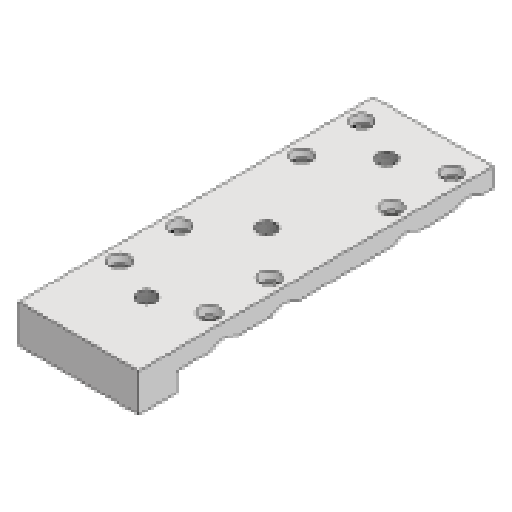
# Autodesk Inventor part: Carrige Attatchment
Saved by Autodesk Inventor 2023 (Build 270158000, 158)
## iProperties
Created: 2022-11-02
Part Number: Carrige Attatchment
Material: Generic
Document SubType Name: Modeling
Designer: deli
Density: 1 g/cm^3
Appearance: Default
Author: deli
Autodesk Inventor part; units mm, degrees
ref_plane "YZ Plane" through (0, 0, 0) normal (1, 0, 0) x (0, 1, 0)
ref_plane "XZ Plane" through (0, 0, 0) normal (0, 1, 0) x (-1, 0, 0)
ref_plane "XY Plane" through (0, 0, 0) normal (0, 0, 1) x (1, 0, 0)
sketch "Sketch1" plane through (0, 0, 0) normal (0, 1, 0) x (-1, 0, 0)
  line L0 (12.8211, 54.4482) -> (-7.1789, 54.4482)
  line L1 (-7.1789, 54.4482) -> (-7.1789, -4.7018)
  line L2 (-7.1789, -4.7018) -> (12.8211, -4.7018)
  line L3 (12.8211, -4.7018) -> (12.8211, 54.4482)
  circle A0 centre (10.3211, 38.6482) radius 1.6
  circle A1 centre (10.3211, 28.6482) radius 1.6
  circle A2 centre (-4.6789, 38.6482) radius 1.6
  circle A3 centre (-4.6789, 28.6482) radius 1.6
  line L4 (10.3211, 38.6482) -> (10.3211, 28.6482) construction
  line L5 (10.3211, 28.6482) -> (-4.6789, 28.6482) construction
  line L6 (-4.6789, 28.6482) -> (-4.6789, 38.6482) construction
  line L7 (-4.6789, 38.6482) -> (10.3211, 38.6482) construction
  circle A4 centre (10.3211, 9.7482) radius 1.6
  circle A5 centre (10.3211, -0.2518) radius 1.6
  circle A6 centre (-4.6789, 9.7482) radius 1.6
  circle A7 centre (-4.6789, -0.2518) radius 1.6
  line L8 (10.3211, 9.7482) -> (10.3211, -0.2518) construction
  line L9 (10.3211, -0.2518) -> (-4.6789, -0.2518) construction
  line L10 (-4.6789, -0.2518) -> (-4.6789, 9.7482) construction
  line L11 (-4.6789, 9.7482) -> (10.3211, 9.7482) construction
  circle A8 centre (2.8211, 43.0982) radius 1.5
  circle A9 centre (2.8211, 23.0982) radius 1.5
  circle A10 centre (2.8211, 3.0982) radius 1.5
  line L12 (2.8211, 43.0982) -> (2.8211, 3.0982) construction
  point P0 (0, 0)
  dimension "d0" = 20
  dimension "d1" = 59.15
  dimension "d2" = 3.2
  dimension "d4" = 10
  dimension "d7" = 15
  dimension "d8" = 2.5
  dimension "d9" = 15.8
  dimension "d10" = 3.2
  dimension "d11" = 10
  dimension "d12" = 15
  dimension "d13" = 2.5
  dimension "d14" = 4.45
  dimension "d15" = 3
  dimension "d18" = 20
  dimension "d19" = 20
  dimension "d25" = 9.85
  dimension "d40" = 10
  constraints: 26 end point, 11 centre point, 8 equal radius, 5 perpendicular, 4 parallel, 3 vertical, 1 horizontal, 1 midpoint
  measures "d0" distance of L2.end L1.end
  measures "d1" distance of L1.end L0.end
  measures "d2" diameter of A0
  measures "d4" distance of L4.end L4.start
  measures "d7" distance of L6.end L4.start
  measures "d8" distance between parallel lines of L3 L4
  measures "d9" distance between parallel lines of L0 L7
  measures "d10" diameter of A4
  measures "d11" distance of L9.start L11.end
  measures "d12" distance of L10.end L11.end
  measures "d13" distance between parallel lines of L3 L8
  measures "d14" distance between parallel lines of L2 L9
  measures "d15" diameter of A8
  measures "d18" distance of A9.centre L12.start
  measures "d19" distance of A9.centre L12.end
  measures "d25" distance edge to line of A8 L0
  measures "d40" distance from line of L1 L12.start
extrude "Extrusion1" add sketch "Sketch1" along normal blind 3.175
chamfer "Chamfer1" distance 1.7 angle 45 8 edges at (-8.7211, 0, 38.6482) (-8.7211, 0, 28.6482) (6.2789, 0, 38.6482) (6.2789, 0, 28.6482) (6.2789, 0, 9.7482) (6.2789, 0, -0.2518) (-8.7211, 0, -0.2518) (-8.7211, 0, 9.7482)
sketch "Sketch2" plane through (0, 0, 0) normal (0, -1, 0) x (1, 0, 0)
  line L0 (-12.8211, 54.4482) -> (7.1789, 54.4482) projected
  line L1 (-12.8211, -4.7018) -> (-12.8211, 54.4482) projected
  line L2 (7.1789, 54.4482) -> (-12.8211, 54.4482)
  line L3 (-12.8211, 54.4482) -> (-12.8211, 48.0982)
  line L4 (-12.8211, 48.0982) -> (7.1789, 48.0982)
  line L5 (7.1789, 48.0982) -> (7.1789, 54.4482)
  point P0 (0, 0)
  dimension "d26" = 6.35
  constraints: 8 end point, 2 parallel, 1 horizontal, 1 perpendicular, 1 point on line
  measures "d26" distance of L3.end L2.end
extrude "Extrusion2" add sketch "Sketch2" along normal blind 3.175
thread "Thread1" size "M3x0.5" class "6H" standard "ANSI Metric M Profile" full length
thread "Thread2" size "M3x0.5" class "6H" standard "ANSI Metric M Profile" full length
thread "Thread3" size "M3x0.5" class "6H" standard "ANSI Metric M Profile" full length
sketch "Sketch4" plane through (-12.8211, 0, -4.7018) normal (-1, 0, 0) x (0, 0, 1)
  line L0 (52.8, -3.175) -> (59.15, -3.175) projected
  line L1 (52.8, -3.175) -> (59.15, 3.175) construction
  circle A0 centre (55.975, 0) radius 1.5
  point P0 (4.7018, 0)
  dimension "d41" = 3
  constraints: 2 end point, 1 centre point, 1 coincident, 1 midpoint
  measures "d41" diameter of A0
extrude "Extrusion4" cut sketch "Sketch4" against normal blind 8
thread "Thread5" size "M3x0.5" class "6H" standard "ANSI Metric M Profile" full length
equation "\"d13\" = d8"
equation "\"d19\" = d18"
equation "\"d40\" = 0.5 * d0"
body "Solid1"
